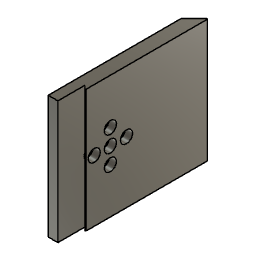
Ofen-Adapterplatte (Autodesk Fusion 360 design; units mm, degrees)
Autodesk Fusion 360 part; units mm, degrees
sketch "Skizze1" plane through (0, 0, 0) normal (0, 0, 1) x (1, 0, 0)
  line L0 (-2.5, 19.7043) -> (-8.5, 19.7043)
  line L1 (-8.5, 19.7043) -> (-8.5, -52.5)
  line L2 (-8.5, -52.5) -> (-2.5, -52.5)
  line L3 (-2.5, -52.5) -> (-2.5, -35.8)
  line L4 (-2.5, -35.8) -> (0, -38.3)
  line L5 (0, -38.3) -> (0, 38.3)
  line L6 (0, 38.3) -> (-2.5, 35.8)
  line L7 (-2.5, 35.8) -> (-2.5, 19.7043)
  line L8 (-2.5, 35.8) -> (-8.5, 29.8)
  line L9 (-8.5, 29.8) -> (-8.5, 19.7043)
  line L10 (-0.5, 37.8) -> (-0.25, 37.8)
  line L11 (-0.25, 37.8) -> (0, 37.55)
  line L12 (0, 0) -> (7.5514, 0) construction
  line L13 (-0.5, -37.8) -> (-0.25, -37.8)
  line L14 (-0.25, -37.8) -> (0, -37.55)
  dimension "d1" = 45
  dimension "d2" = 2.5
  dimension "d6" = 52.5
  dimension "d31" = 8.5
  dimension "d33" = 16.7
  dimension "d34" = 0.25
  dimension "d36" = 0.25
  dimension "d37" = 82.3
  constraint horizontal L0
  constraint perpendicular L0 L1
  constraint perpendicular L1 L2
  constraint perpendicular L2 L3
  constraint perpendicular L2 L5
  constraint perpendicular L4 L6
  constraint perpendicular L0 L7
  constraint collinear L3 L7
  constraint parallel L6 L8
  constraint parallel L7 L9
  constraint midpoint L5 L12.start
  constraint coincident L12.start origin
  constraint horizontal L10
  constraint coincident L5 L11.end
  constraint perpendicular L6 L11
  constraint coincident L6 L10.start
  constraint perpendicular L5 L12
  constraint symmetric L10.start L12 L13.start
  constraint symmetric L10.end L12 L13.end
  constraint symmetric L11.end L12 L14.end
  measures "d1" angle of L3 L4
  measures "d2" distance of L3.end L5
  measures "d6" distance of L2 L12.start
  measures "d31" distance of L1 L5
  measures "d33" distance of L2.end L3.end
  measures "d34" distance of L13.start L13.end
  measures "d36" horizontal distance of L13.end L14.end
  measures "d37" distance of L1.end L8.end
extrude "Extrusion1" add sketch "Skizze1" along normal blind 76 contours L0 L1 L2 L3 L4 L5 L6 L7 L10 L11 L13 L14 | L0 L7 L8 L9
sketch "Skizze2" plane through (0, 0, 0) normal (1, 0, 0) x (0, 1, 0)
  line L0 (-37.55, 0) -> (37.55, 0)
  line L1 (37.55, 76) -> (-37.55, 76)
  line L2 (0, 38) -> (-32.5, 38) construction
  circle A0 centre (-12.5, 38) radius 2
  circle A1 centre (-32.5, 38) radius 2
  circle A2 centre (-22.5, 48) radius 2
  circle A3 centre (-22.5, 28) radius 2
  line L3 (-32.5, 38) -> (-12.5, 38) construction
  line L4 (-22.5, 38) -> (-22.5, 48) construction
  circle A4 centre (-22.5, 38) radius 2
  circle A5 centre (-12.5, 38) radius 3.75
  circle A6 centre (-22.5, 48) radius 3.75
  circle A7 centre (-22.5, 28) radius 3.75
  circle A8 centre (-32.5, 38) radius 3.75
  circle A9 centre (-22.5, 38) radius 3.75
  line L5 (37.55, 0) -> (37.55, 76)
  line L6 (-37.55, 76) -> (-37.55, 0)
  line L7 (0, 76) -> (0, 0) construction
  dimension "d9" = 4
  dimension "d11" = 4
  dimension "d12" = 4
  dimension "d13" = 4
  dimension "d14" = 20
  dimension "d15" = 10
  dimension "d16" = 4
  dimension "d19" = 7.5
  dimension "d20" = 7.5
  dimension "d21" = 7.5
  dimension "d22" = 7.5
  dimension "d23" = 7.5
  dimension "d32" = 12.5
  constraint coincident L2 A0.centre
  constraint coincident L2 A1.centre
  constraint coincident L2.end A1.centre
  constraint coincident A0.centre L3.end
  constraint midpoint L3 L4.start
  constraint coincident A2.centre L4.end
  constraint perpendicular L3 L4
  constraint symmetric A2.centre A3.centre L3
  constraint coincident L4.start A4.centre
  constraint concentric A0 A5
  constraint concentric A2 A6
  constraint concentric A3 A7
  constraint concentric A1 A8
  constraint concentric A4 A9
  constraint midpoint L1 L7.start
  constraint coincident L7.end origin
  constraint midpoint L2.start L7
  constraint horizontal L2
  measures "d9" diameter of A0
  measures "d11" diameter of A1
  measures "d12" diameter of A2
  measures "d13" diameter of A3
  measures "d14" distance of A0.centre L2.end
  measures "d15" distance of L4.start A2.centre
  measures "d16" diameter of A4
  measures "d19" diameter of A5
  measures "d20" diameter of A6
  measures "d21" diameter of A7
  measures "d22" diameter of A8
  measures "d23" diameter of A9
  measures "d32" distance of L2.start A0.centre
extrude "Extrusion3" cut sketch "Skizze2" against normal blind 4.5 contours A5 | A6 | A7 | A8 | A9
extrude "Extrusion2" cut sketch "Skizze2" against normal up to surface (8.5 mm away) contours A0 | A1 | A2 | A3 | A4
equation "d6 = 12.5 mm + 20 mm + 20 mm"
equation "d11 = d9"
equation "d12 = d9"
equation "d13 = d9"
equation "d16 = d9"
equation "d20 = d19"
equation "d21 = d19"
equation "d22 = d19"
equation "d23 = d19"
